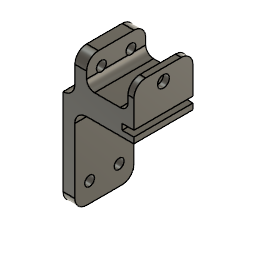
ISO 6 (Autodesk Fusion 360 design; units mm, degrees)
part number: 2025-12-18-11-41-26-592
Autodesk Fusion 360 part; units mm, degrees
sketch "Sketch1" plane through (0, 0, 0) normal (0, 1, 0) x (1, 0, 0)
  line L0 (0, 0) -> (0, -100)
  line L1 (12, -112) -> (12, -142)
  arc A0 (12, -112) -> (0, -100) centre (0, -112) ccw
  line L2 (12, -142) -> (24, -142)
  line L3 (0, 0) -> (12, 0)
  line L4 (12, 0) -> (12, -78)
  line L5 (24, -90) -> (72, -90)
  line L6 (32, -115) -> (58, -115)
  line L7 (24, -142) -> (24, -123)
  arc A1 (32, -115) -> (24, -123) centre (32, -123) ccw
  line L8 (66, -142) -> (66, -123)
  arc A2 (66, -123) -> (58, -115) centre (58, -123) ccw
  line L9 (66, -142) -> (72, -142)
  line L10 (72, -142) -> (72, -90)
  arc A3 (12, -78) -> (24, -90) centre (24, -78) ccw
  point P0 (12, -90)
  dimension "d1" = 100
  dimension "d2" = 24
  dimension "d4" = 142
  dimension "d6" = 12
  dimension "d7" = 90
  dimension "d8" = 25
  dimension "d9" = 8
  dimension "d10" = 42
  dimension "d11" = 8
  dimension "d12" = 6
  dimension "d13" = 12
  constraint coincident L0.start L3.start
  constraint vertical L0
  constraint tangent L1 A0
  constraint vertical L0.end A0.centre
  constraint perpendicular L1 L2
  constraint perpendicular L0 L3
  constraint perpendicular L3 L4
  constraint perpendicular L4 L5
  constraint perpendicular L1 L6
  constraint perpendicular L6 L7
  constraint tangent L7 A1
  constraint tangent L6 A1
  constraint perpendicular L5 L8
  constraint tangent L6 A2
  constraint tangent L8 A2
  constraint horizontal L2.end L8.start
  constraint perpendicular L8 L9
  constraint perpendicular L5 L10
  constraint coincident P0 L4
  constraint coincident P0 L5
  constraint tangent L4 A3
  constraint tangent L5 A3
  measures "d1" distance of L0.start L0.end
  measures "d2" diameter of A0
  measures "d4" vertical distance of L0.start L1.end
  measures "d6" distance of L0.start L3.end
  measures "d7" distance of L3.end P0
  measures "d8" distance of L5 L6
  measures "d9" radius of A1
  measures "d10" distance of L7 L8
  measures "d11" radius of A2
  measures "d12" distance of L8.start L9.end
  measures "d13" radius of A3
extrude "Extrude1" add sketch "Sketch1" along normal blind 60
fillet "Fillet1" radius 12 2 edges at (18, 60, 142) (18, 0, 142)
fillet "Fillet2" radius 12 2 edges at (69, 0, 142) (69, 60, 142)
fillet "Fillet3" radius 12 2 edges at (6, 60, 0) (6, 0, 0)
sketch "Sketch2" plane through (0, 0, 0) normal (0, -1, 0) x (1, 0, 0)
  line L0 (0, 12) -> (12, 12)
  line L1 (12, 12) -> (12, 78)
  arc A0 (24, 90) -> (12, 78) centre (24, 78) ccw
  line L2 (24, 90) -> (72, 90)
  line L3 (72, 90) -> (72, 130)
  line L4 (72, 130) -> (66, 130)
  line L5 (66, 130) -> (66, 123)
  arc A1 (58, 115) -> (66, 123) centre (58, 123) ccw
  line L6 (58, 115) -> (32, 115)
  arc A2 (24, 123) -> (32, 115) centre (32, 123) ccw
  line L7 (24, 123) -> (24, 130)
  line L8 (24, 130) -> (12, 130)
  line L9 (12, 130) -> (12, 112)
  arc A3 (0, 100) -> (12, 112) centre (0, 112) ccw
  line L10 (0, 100) -> (0, 12)
  line L11 (60, 102) -> (72, 102)
  line L12 (72, 102) -> (72, 96)
  line L13 (72, 96) -> (60, 96)
  line L14 (60, 96) -> (60, 102)
  dimension "d22" = 6
  dimension "d23" = 12
  dimension "d24" = 12
  constraint horizontal L11
  constraint vertical L12
  constraint horizontal L13
  constraint vertical L14
  constraint coincident L2.end L12
  measures "d22" distance of L2 L13
  measures "d23" distance of L11.start L11.end
  measures "d24" distance of L2 L11
extrude "Extrude2" cut sketch "Sketch2" against normal through all contours L3 L11 L12 L13 L14
sketch "Sketch3" plane through (72, 0, 0) normal (1, 0, 0) x (0, 1, 0)
  line L0 (0, 102) -> (60, 102)
  line L1 (60, 102) -> (60, 130)
  arc A0 (60, 130) -> (48, 142) centre (48, 130) ccw
  line L2 (48, 142) -> (12, 142)
  arc A1 (12, 142) -> (0, 130) centre (12, 130) ccw
  line L3 (0, 130) -> (0, 102)
  point P0 (30, 130)
hole "Hole1" at (72, 30, 130) direction (-1, 0, 0) diameter 12 depth 6 tip angle 118
sketch "Sketch4" plane through (12, 0, 0) normal (1, 0, 0) x (0, 1, 0)
  arc A0 (0, 12) -> (12, 0) centre (12, 12) ccw
  line L0 (12, 0) -> (48, 0)
  arc A1 (48, 0) -> (60, 12) centre (48, 12) ccw
  line L1 (60, 12) -> (60, 78)
  line L2 (60, 78) -> (0, 78)
  line L3 (0, 78) -> (0, 12)
  point P0 (15, 20)
  point P1 (45, 20)
  dimension "d30" = 15
  dimension "d31" = 15
  dimension "d32" = 20
  measures "d30" distance of L3 P0
  measures "d31" distance of L1 P1
  measures "d32" distance of L0 P1
hole "Hole2" at (12, 45, 20) at (12, 15, 20) direction (-1, 0, 0) diameter 10 depth 12 tip angle 118
sketch "Sketch5" plane through (12, 0, 0) normal (-1, 0, 0) x (0, -1, 0)
  arc A0 (0, 130) -> (-12, 142) centre (-12, 130) ccw
  line L0 (-12, 142) -> (-48, 142)
  arc A1 (-48, 142) -> (-60, 130) centre (-48, 130) ccw
  line L1 (-60, 130) -> (-60, 112)
  line L2 (-60, 112) -> (0, 112)
  line L3 (0, 112) -> (0, 130)
  point P0 (-45, 127)
  point P1 (-15, 127)
  dimension "d36" = 30
  dimension "d37" = 15
  dimension "d38" = 15
  measures "d36" distance of P0 P1
  measures "d37" distance of L0 P0
  measures "d38" distance of L1 P0
hole "Hole3" at (12, 45, 127) at (12, 15, 127) direction (1, 0, 0) diameter 10 depth 12 tip angle 118
